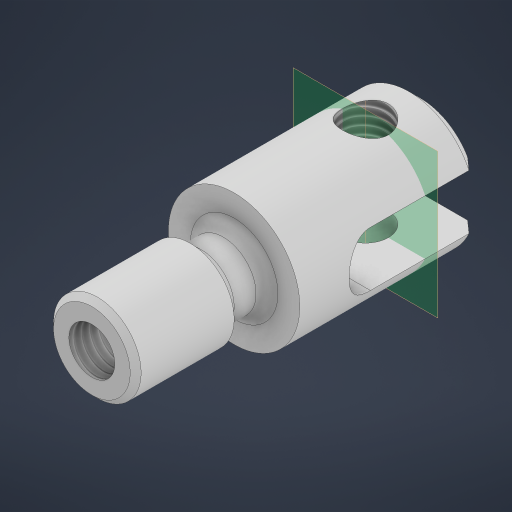
# Autodesk Inventor part: Part1
Saved by Autodesk Inventor 2023 (Build 270158000, 158)
## iProperties
Created: 2022-11-27
Part Number: Part1
Material: Generic
Document SubType Name: Modeling
Designer: iusti
Density: 1 g/cm^3
Appearance: Default
Author: iusti
Autodesk Inventor part; units mm, degrees
ref_plane "XZ Plane" through (0, 0, 0) normal (0, 1, 0) x (-1, 0, 0)
ref_plane "XY Plane" through (0, 0, 0) normal (0, 0, 1) x (1, 0, 0)
sketch "Sketch1" plane through (0, 0, 0) normal (1, 0, 0) x (0, 1, 0)
  line L0 (0, 67.4997) -> (0, -67.4997)
  line L1 (0, 60) -> (8, 60)
  line L2 (8, 60) -> (8, 42)
  line L3 (8, 42) -> (6, 42)
  line L4 (6, 42) -> (6, 34)
  line L5 (6, 34) -> (12, 34)
  line L6 (12, 34) -> (12, 0)
  line L7 (12, 0) -> (0, 0)
  dimension "d0" = 24
  dimension "d1" = 60
  dimension "d2" = 18
  dimension "d3" = 16
  dimension "d4" = 12
  dimension "d5" = 26
  constraints: 16 end point, 7 perpendicular, 1 coincident, 1 midpoint, 1 point on line, 1 vertical
  measures "d0" diameter of L6 L0
  measures "d1" distance between parallel lines of L1 L7
  measures "d2" distance of L1.end L2.end
  measures "d3" diameter of L2 L0
  measures "d4" diameter of L4 L0
  measures "d5" distance between parallel lines of L5 L1
revolve "Revolution1" add sketch "Sketch1" angle 360 about axis through (0, 0, 67.4997) along (0, 0, -1)
chamfer "Chamfer1" distance 1 angle 45 1 edges at (0, -8, 60)
chamfer "Chamfer2" distance 2 angle 45 1 edges at (0, -12, 0)
fillet "Fillet1" radius 2 2 edges at (0, -6, 42) (0, -6, 34)
sketch "Sketch2" plane through (0, 0, 60) normal (0, 0, 1) x (1, 0, 0)
  circle A0 centre (0, 0) radius 7 projected
  point P0 (0, 0)
  constraints: 1 coincident
hole "Hole1" at (0, 0, 60) direction (0, 0, -1) diameter 8.376 depth 22 tip angle 118 thread size "M10x1.5" class "6H" standard "ISO Metric profile"
sketch "Sketch3" plane through (0, 0, 0) normal (1, 0, 0) x (0, 1, 0)
  line L0 (10, 0) -> (-10, 0) projected
  line L1 (5, 0) -> (5, 20)
  arc A0 (5, 20) -> (-5, 20) centre (0, 20) ccw
  line L2 (-5, 20) -> (-5, 0)
  line L3 (-5, 0) -> (5, 0)
  point P0 (0, 0)
  dimension "d21" = 10
  dimension "d22" = 20
  constraints: 6 end point, 2 point on circle, 2 point on line, 2 tangent, 2 vertical, 1 centre point, 1 midpoint, 1 perpendicular
  measures "d21" distance between parallel lines of L2 L1
  measures "d22" distance from line of L0 A0.centre
extrude "Extrusion1" cut sketch "Sketch3" along normal through all both and the other way through all
hole "Hole3" at (0, 12, 10) direction (0, -1, 0) diameter 8.376 end through all thread size "M10x1.5" class "6H" standard "ISO Metric profile"
ref_plane "Work Plane2" through (0, 0, 10) normal (0, 0, -1) x (-1, 0, 0)
equation "\"d38\" = 0.5 * d5"
body "Solid1"
